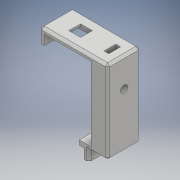
# Autodesk Inventor part: FEMUR2_B
Saved by Autodesk Inventor 2017 (Build 210142000, 142)
## iProperties
Created: 2017-09-24
Part Number: FEMUR2_B
Material: Generic
Document SubType Name: Modeling
Designer: Alexander Miller
Density: 1 g/cm^3
Appearance: Default
Author: Alexander Miller
Autodesk Inventor part; units mm, degrees
ref_plane "YZ Plane" through (0, 0, 0) normal (1, 0, 0) x (0, 1, 0)
ref_plane "XZ Plane" through (0, 0, 0) normal (0, 1, 0) x (-1, 0, 0)
ref_plane "XY Plane" through (0, 0, 0) normal (0, 0, 1) x (1, 0, 0)
sketch "Sketch1" plane through (0, 0, 0) normal (0, 1, 0) x (-1, 0, 0)
  line L0 (23.7482, 13.5362) -> (23.7482, 19.7862)
  line L1 (23.7482, 19.7862) -> (-5.2518, 19.7862)
  line L2 (-5.2518, 19.7862) -> (-5.2518, -15.7138)
  line L3 (-5.2518, -15.7138) -> (2.7482, -15.7138)
  line L4 (2.7482, -15.7138) -> (2.7482, -19.9638)
  line L5 (2.7482, -19.9638) -> (4.7482, -19.9638)
  line L6 (6.7482, -13.7138) -> (-1.2518, -13.7138)
  line L7 (-1.2518, -13.7138) -> (-1.2518, 17.7862)
  line L8 (-1.2518, 17.7862) -> (21.7482, 17.7862)
  line L9 (21.7482, 17.7862) -> (21.7482, 13.5362)
  line L10 (21.7482, 13.5362) -> (23.7482, 13.5362)
  line L11 (6.7482, -13.7138) -> (6.7482, -15.7138)
  line L12 (6.7482, -15.7138) -> (4.7482, -15.7138)
  line L13 (4.7482, -15.7138) -> (4.7482, -19.9638)
  point P0 (0, 0)
  dimension "d1" = 4.25
  dimension "d2" = 2
  dimension "d3" = 2
  dimension "d4" = 2
  dimension "d5" = 2
  dimension "d6" = 4
  dimension "d7" = 23
  dimension "d8" = 2
  dimension "d9" = 4.25
  dimension "d10" = 2
  dimension "d21" = 31.5
  dimension "d22" = 8
  constraints: 28 end point, 11 perpendicular, 2 vertical
  measures "d1" distance of L8.end L9.end
  measures "d2" distance of L9.end L0.start
  measures "d3" distance of L4.end L5.end
  measures "d4" distance between parallel lines of L6 L3
  measures "d5" distance between parallel lines of L8 L1
  measures "d6" distance between parallel lines of L2 L7
  measures "d7" distance of L7.end L8.end
  measures "d8" distance of L11.end L12.end
  measures "d9" distance of L12.end L5.end
  measures "d10" distance of L6.start L11.end
  measures "d21" distance between parallel lines of L8 L6
  measures "d22" distance between parallel lines of L7 L11
extrude "Extrusion1" add sketch "Sketch1" along normal blind 14
sketch "Sketch2" plane through (-23.7482, 0, 13.5362) normal (-1, 0, 0) x (0, 0, 1)
  circle A0 centre (2.5, 7) radius 1
  line L0 (6.25, 0) -> (6.25, 14) projected
  line L1 (0, 0) -> (0, 14) projected
  point P0 (-13.5362, 0)
  point P1 (6.25, 7)
  dimension "d13" = 1.5
  dimension "d14" = 2
  constraints: 1 centre point, 1 horizontal alignment, 1 midpoint
  measures "d13" distance edge to line of A0 L1
  measures "d14" diameter of A0
extrude "Extrusion2" cut sketch "Sketch2" against normal up to surface (2 mm away)
sketch "Sketch3" plane through (-4.7482, 0, -19.9638) normal (-1, 0, 0) x (0, 0, 1)
  circle A0 centre (2.5, 7) radius 1
  line L0 (0, 0) -> (0, 14) projected
  point P0 (19.9638, 0)
  point P1 (0, 7)
  dimension "d17" = 1.5
  dimension "d18" = 2
  constraints: 1 centre point, 1 horizontal alignment, 1 midpoint
  measures "d17" distance edge to line of A0 L0
  measures "d18" diameter of A0
extrude "Extrusion3" cut sketch "Sketch3" against normal up to surface (2 mm away)
chamfer "Chamfer1" distance 1 angle 45 13 edges at (5.2518, 0, 2.0362) (5.2518, 14, 2.0362) (-9.2482, 14, 19.7862) (-9.2482, 0, 19.7862) (-23.7482, 0, 16.6612) (-23.7482, 14, 16.6612) (-23.7482, 7, 19.7862) (5.2518, 7, -15.7138) (1.2518, 14, -15.7138) (1.2518, 0, -15.7138) (-2.7482, 14, -17.8388) (-2.7482, 0, -17.8388) (5.2518, 7, 19.7862)
sketch "Sketch4" plane through (5.2518, 1, -14.7138) normal (1, 0, 0) x (0, 0, -1)
  circle A0 centre (2.75, 6) radius 2.5
  circle A1 centre (2.75, 6) radius 1 projected
  point P0 (-14.7138, -1)
  dimension "d26" = 5
  constraints: 1 centre point, 1 concentric
  measures "d26" diameter of A0
extrude "Extrusion4" cut sketch "Sketch4" against normal up to surface (8 mm away) contours A0 | A1
sketch "Sketch5" plane through (-22.7482, 1, 19.7862) normal (0, 0, 1) x (1, 0, 0)
  line L0 (24, -1) -> (24, 13) projected
  line L1 (22, 8.5) -> (24, 8.5)
  line L2 (24, 8.5) -> (24, 3.5)
  line L3 (24, 3.5) -> (22, 3.5)
  line L4 (22, 3.5) -> (22, 8.5)
  point P0 (22.7482, -1)
  point P1 (24, 6)
  point P2 (24, 6)
  dimension "d29" = 2
  dimension "d30" = 5
  constraints: 8 end point, 2 midpoint, 2 parallel, 1 coincident, 1 collinear, 1 horizontal, 1 perpendicular
  measures "d29" distance of L1.start L1.end
  measures "d30" distance of L3.end L1.start
extrude "Extrusion5" cut sketch "Sketch5" against normal up to surface (2 mm away)
sketch "Sketch8" plane through (-22.7482, 1, 19.7862) normal (0, 0, 1) x (1, 0, 0)
  line L0 (1, -1) -> (1, 13) projected
  line L1 (7, 8.5) -> (12, 8.5)
  line L2 (12, 8.5) -> (12, 3.5)
  line L3 (12, 3.5) -> (7, 3.5)
  line L4 (7, 3.5) -> (7, 8.5)
  line L5 (22, 3.5) -> (22, 8.5) projected
  line L6 (3, 11.0075) -> (16, 11.0075) construction
  line L7 (16, 11.0075) -> (16, 0.9925) construction
  line L8 (16, 0.9925) -> (3, 0.9925) construction
  line L9 (3, 0.9925) -> (3, 11.0075) construction
  point P0 (22.7482, -1)
  point P1 (3, 6)
  point P2 (1, 6)
  point P3 (7, 6)
  point P4 (9.5, 11.0075)
  point P5 (9.5, 8.5)
  dimension "d39" = 5
  dimension "d40" = 13
  dimension "d43" = 2
  constraints: 16 end point, 5 midpoint, 5 parallel, 2 horizontal, 2 horizontal alignment, 2 perpendicular, 1 vertical alignment
  measures "d39" distance of L1.start L1.end
  measures "d40" distance of L6.start L6.end
  measures "d43" distance between parallel lines of L0 L9
extrude "Extrusion8" cut sketch "Sketch8" against normal up to surface (2 mm away)
sketch "Sketch9" plane through (1.2518, 0, -13.7138) normal (-1, 0, 0) x (0, 0, 1)
  line L0 (0, 14) -> (31.5, 14)
  line L1 (31.5, 14) -> (31.5, 13)
  line L2 (31.5, 13) -> (0, 13)
  line L3 (0, 13) -> (0, 14)
  line L4 (0, 1) -> (31.5, 1)
  line L5 (31.5, 1) -> (31.5, 0)
  line L6 (31.5, 0) -> (0, 0)
  line L7 (0, 0) -> (0, 1)
  line L8 (0, 14) -> (31.5, 14) projected
  line L9 (0, 0) -> (31.5, 0) projected
  line L10 (31.5, 0) -> (31.5, 4.5) projected
  line L11 (31.5, 9.5) -> (31.5, 14) projected
  line L12 (0, 0) -> (0, 14) projected
  point P0 (13.7138, 0)
  dimension "d44" = 1
  constraints: 16 end point, 7 collinear, 4 parallel, 2 horizontal, 2 perpendicular
  measures "d44" distance of L0.end L1.end
extrude "Extrusion9" add sketch "Sketch9" along normal blind 3
sketch "Sketch6" plane through (5.2518, 1, -14.7138) normal (1, 0, 0) x (0, 0, -1)
  line L0 (-28.25, -1) -> (-28.25, 13) projected
  circle A0 centre (-22.25, 6) radius 6
  circle A1 centre (-22.25, 6) radius 1.5
  line L1 (-32.5, 12) -> (-1, 12) projected
  line L2 (-1, 0) -> (-32.5, 0) projected
  point P0 (-14.7138, -1)
  dimension "d33" = 3
  constraints: 3 tangent, 2 centre point, 1 coincident
  measures "d33" diameter of A1
extrude "Extrusion6" cut sketch "Sketch6" against normal up to surface (4 mm away) contours A1
sketch "Sketch7" plane through (1.2518, 0, -13.7138) normal (-1, 0, 0) x (0, 0, 1)
  line L0 (24, 4.25) -> (18.5, 4.25)
  line L1 (18.5, 4.25) -> (18.5, 9.75)
  line L2 (18.5, 9.75) -> (24, 9.75)
  line L3 (24, 9.75) -> (24, 4.25)
  circle A0 centre (21.25, 7) radius 1.5 projected
  point P0 (13.7138, 0)
  point P1 (21.25, 4.25)
  point P2 (24, 7)
  dimension "d36" = 5.5
  constraints: 8 end point, 2 midpoint, 2 parallel, 2 perpendicular, 1 horizontal, 1 horizontal alignment, 1 vertical alignment
  measures "d36" distance of L0.start L0.end
extrude "Extrusion7" cut sketch "Sketch7" against normal blind 1.8
sketch "Sketch10" plane through (-21.7482, 0, 17.7862) normal (0, 0, -1) x (-1, 0, 0)
  line L0 (-6, 4.5) -> (-4, 4.5)
  line L1 (-4, 4.5) -> (-4, 9.5)
  line L2 (-4, 9.5) -> (-6, 9.5)
  line L3 (-6, 9.5) -> (-6, 4.5)
  line L4 (-6, 9.5) -> (-6, 4.5) projected
  line L5 (-11, 9.5) -> (-6, 9.5) projected
  line L6 (-6, 4.5) -> (-11, 4.5) projected
  point P0 (-21.7482, 0)
  dimension "d47" = 2
  constraints: 8 end point, 3 collinear, 2 parallel, 1 horizontal, 1 perpendicular
  measures "d47" distance of L1.end L2.end
extrude "Extrusion10" cut sketch "Sketch10" against normal blind 1
equation "\"d1\" = -0.5 * servo_A + 0.5 * servo_D"
equation "\"d7\" = servo_E + servo_F"
equation "\"d8\" = servo_F"
equation "\"d9\" = -0.5 * servo_A + 0.5 * servo_D"
equation "\"d21\" = servo_D"
equation "\"d13\" = servo_L"
equation "\"d14\" = servo_H"
equation "\"d15\" = servo_B"
equation "\"d17\" = servo_L"
equation "\"d18\" = servo_H"
equation "\"d19\" = servo_B"
equation "\"d30\" = servo_K"
equation "\"d39\" = servo_K"
equation "\"d43\" = servo_F"
equation "\"d41\" = nut_C"
equation "\"d33\" = bearing_B"
equation "\"d36\" = nut_A"
equation "\"d37\" = nut_B"
equation "\"servo_A\" = 23"
equation "\"servo_D\" = 31.5"
equation "\"servo_E\" = 21"
equation "\"servo_F\" = 2"
equation "\"servo_L\" = 1.5"
equation "\"servo_H\" = 2"
equation "\"servo_B\" = 12"
equation "\"servo_K\" = 5"
equation "\"nut_C\" = 3"
equation "\"bearing_B\" = 3"
equation "\"nut_A\" = 5.5"
equation "\"nut_B\" = 1.8"
body "Solid1"
